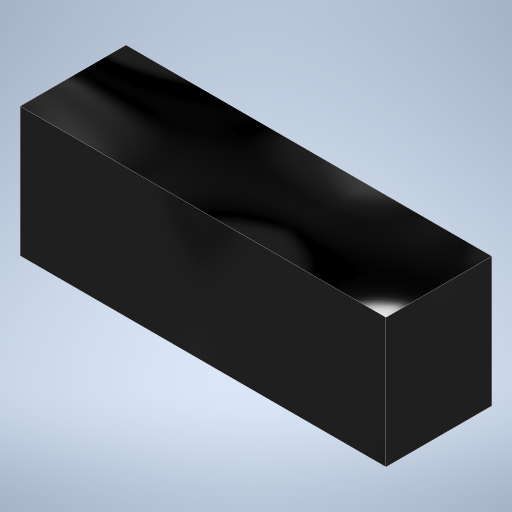
# Autodesk Inventor part: magnet
Saved by Autodesk Inventor 2023 (Build 270158000, 158)
## iProperties
Created: 2023-04-11
Part Number: magnet
Material: Generic
Document SubType Name: Modeling
Designer: Sam
Density: 1 g/cm^3
Appearance: Default
Author: Sam
Autodesk Inventor part; units mm, degrees
ref_plane "YZ Plane" through (0, 0, 0) normal (1, 0, 0) x (0, 1, 0)
ref_plane "XZ Plane" through (0, 0, 0) normal (0, 1, 0) x (-1, 0, 0)
ref_plane "XY Plane" through (0, 0, 0) normal (0, 0, 1) x (1, 0, 0)
sketch "Sketch1" plane through (0, 0, 0) normal (0, 1, 0) x (-1, 0, 0)
  line L0 (-4.9149, 1.4224) -> (4.9149, 1.4224)
  line L1 (4.9149, 1.4224) -> (4.9149, -1.4224)
  line L2 (4.9149, -1.4224) -> (-4.9149, -1.4224)
  line L3 (-4.9149, -1.4224) -> (-4.9149, 1.4224)
  line L4 (-4.9149, 1.4224) -> (4.9149, -1.4224) construction
  line L5 (4.9149, 1.4224) -> (-4.9149, -1.4224) construction
  point P0 (0, 0)
  dimension "d0" = 9.8298
  dimension "d1" = 2.8448
  constraints: 12 end point, 2 midpoint, 2 parallel, 1 horizontal, 1 perpendicular
  measures "d0" distance of L0.start L0.end
  measures "d1" distance of L0.end L1.end
extrude "Extrusion1" add sketch "Sketch1" along normal mid plane 3.4798
body "Solid1"
